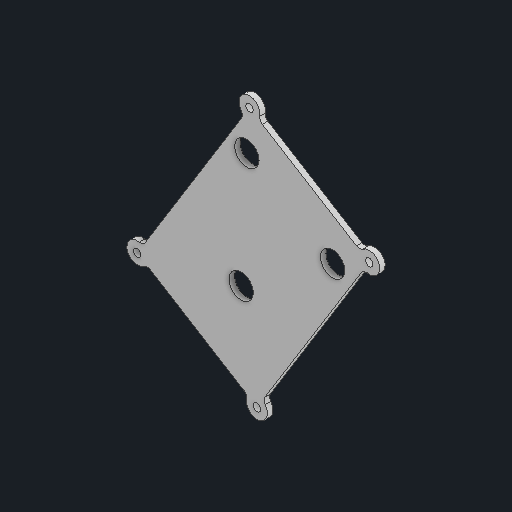
# Autodesk Inventor part: Upper_Plate
Saved by Autodesk Inventor 2024.2 (Build 282272000, 272)
## iProperties
Created: 2024-03-30
Part Number: Upper_Plate
Material: Generic
Document SubType Name: Modeling
Designer: warm
Density: 1 g/cm^3
Appearance: Default
Author: warm
Autodesk Inventor part; units mm, degrees
ref_plane "YZ Plane" through (0, 0, 0) normal (1, 0, 0) x (0, 1, 0)
ref_plane "XZ Plane" through (0, 0, 0) normal (0, 1, 0) x (-1, 0, 0)
ref_plane "XY Plane" through (0, 0, 0) normal (0, 0, 1) x (1, 0, 0)
sketch "Sketch1" plane through (0, 0, 0) normal (0, 0, 1) x (1, 0, 0)
  circle A0 centre (0, 0) radius 7 projected
  circle A1 centre (52.2854, 37.1495) radius 7 projected
  circle A2 centre (3.2487, 67.4218) radius 7 projected
  circle A3 centre (73.2479, 48.3549) radius 2.15
  circle A4 centre (73.9366, 30.5749) radius 3.15 construction
  circle A5 centre (58.8599, 58.8007) radius 3.15 construction
  circle A6 centre (4.7755, 90.6548) radius 2.15
  circle A7 centre (-59.4554, -13.318) radius 2.15
  circle A8 centre (9.0171, -55.618) radius 2.15
  circle A9 centre (38.0853, -27.4589) radius 3.15 construction
  circle A10 centre (-27.4589, -38.0853) radius 3.5 construction
  line L0 (38.0853, -27.4589) -> (9.0171, -55.618) construction
  line L1 (9.0171, -55.618) -> (-27.4589, -38.0853) construction
  line L2 (9.0171, -55.618) -> (73.2479, 48.3549)
  line L3 (92.2333, 46.5881) -> (17.5545, -74.2973) construction
  line L4 (-27.4589, -38.0853) -> (-59.4554, -13.318) construction
  line L5 (-59.4554, -13.318) -> (-42.6755, 23.5008) construction
  line L6 (-59.4554, -13.318) -> (4.7755, 90.6548)
  line L7 (4.7755, 90.6548) -> (73.2479, 48.3549)
  line L8 (9.0171, -55.618) -> (-59.4554, -13.318)
  circle A11 centre (9.0171, -55.618) radius 6
  circle A12 centre (-59.4554, -13.318) radius 6
  circle A13 centre (4.7755, 90.6548) radius 6
  circle A14 centre (73.2479, 48.3549) radius 6
  point P0 (0, 0)
  point P1 (3.9125, -52.4646)
  point P2 (12.1704, -50.5134)
  point P3 (70.0945, 43.2504)
  point P4 (68.1434, 51.5083)
  point P5 (9.88, 87.5015)
  point P6 (1.6221, 85.5503)
  point P7 (-56.302, -8.2135)
  point P8 (-54.3509, -16.4714)
  point P9 (71.4188, 49.4849)
  point P10 (72.118, 46.5258)
  point P11 (3.6455, 88.8257)
  point P12 (6.6046, 89.5249)
  point P13 (-57.6263, -14.448)
  point P14 (-58.3254, -11.4889)
  point P15 (10.147, -53.7888)
  point P16 (7.1879, -54.488)
  dimension "d0" = 4.3
  dimension "d1" = 17.78
  dimension "d2" = 17.78
  dimension "d3" = 4.3
  dimension "d4" = 4.3
  dimension "d5" = 4.3
  dimension "d6" = 40.4622
  dimension "d7" = 12
  dimension "d8" = 12
  dimension "d9" = 12
  dimension "d10" = 12
  constraints: 16 end point, 8 centre point, 4 coincident, 3 parallel, 2 equal length, 1 perpendicular
  measures "d0" diameter of A3
  measures "d1" vertical distance of L2.end A4.centre
  measures "d2" distance of A5.centre L2.end
  measures "d3" diameter of A6
  measures "d4" diameter of A7
  measures "d5" diameter of A8
  measures "d6" distance of L1.end L4.end
  measures "d7" diameter of A11
  measures "d8" diameter of A12
  measures "d9" diameter of A13
  measures "d10" diameter of A14
extrude "Extrusion1" add sketch "Sketch1" along normal blind 3.175 contours A3 L7 A14 L2 | A3 L2 A14 L7 | A14 L2 A11 L8 A12 L6 A13 L7 | A13 L6 A6 L7 | L7 A6 L6 A13 | A11 L8 A8 L2 | L2 A8 L8 A11 | A12 L8 A7 L6 | L6 A7 L8 A12
fillet "Fillet1" radius 3.175 8 edges at (3.9125, -52.4646, 1.5875) (-54.3509, -16.4714, 1.5875) (-56.302, -8.2135, 1.5875) (1.6221, 85.5503, 1.5875) (9.88, 87.5015, 1.5875) (68.1434, 51.5083, 1.5875) (70.0945, 43.2504, 1.5875) (12.1704, -50.5134, 1.5875)
body "Solid1"
